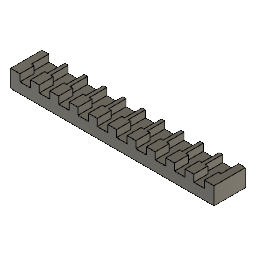
CClampRack3and4in v6 (Autodesk Fusion 360 design; units mm, degrees)
Autodesk Fusion 360 part; units mm, degrees
sketch "Sketch1" plane through (0, 0, 0) normal (0, 0, 1) x (1, 0, 0)
  line L0 (0, 57.15) -> (0, 0)
  line L1 (12.7, 57.15) -> (41.275, 57.15)
  line L2 (41.275, 57.15) -> (41.275, 25.4)
  line L3 (41.275, 25.4) -> (12.7, 25.4)
  line L4 (12.7, 25.4) -> (12.7, 57.15)
  line L5 (26.9875, 25.4) -> (26.9875, 0) construction
  line L6 (17.4625, 25.4) -> (17.4625, 0)
  line L7 (36.5125, 25.4) -> (36.5125, 0)
  line L8 (17.4625, 0) -> (36.5125, 0)
  line L9 (52.3875, 25.4) -> (52.3875, 0)
  line L10 (47.625, 57.15) -> (76.2, 57.15)
  line L11 (61.9125, 25.4) -> (61.9125, 0) construction
  line L12 (47.625, 25.4) -> (47.625, 57.15)
  line L13 (76.2, 25.4) -> (47.625, 25.4)
  line L14 (76.2, 57.15) -> (76.2, 25.4)
  line L15 (71.4375, 25.4) -> (71.4375, 0)
  line L16 (52.3875, 0) -> (71.4375, 0)
  line L17 (87.3125, 25.4) -> (87.3125, 0)
  line L18 (82.55, 57.15) -> (111.125, 57.15)
  line L19 (96.8375, 25.4) -> (96.8375, 0) construction
  line L20 (82.55, 25.4) -> (82.55, 57.15)
  line L21 (111.125, 25.4) -> (82.55, 25.4)
  line L22 (111.125, 57.15) -> (111.125, 25.4)
  line L23 (106.3625, 25.4) -> (106.3625, 0)
  line L24 (87.3125, 0) -> (106.3625, 0)
  line L25 (122.2375, 25.4) -> (122.2375, 0)
  line L26 (117.475, 57.15) -> (146.05, 57.15)
  line L27 (131.7625, 25.4) -> (131.7625, 0) construction
  line L28 (117.475, 25.4) -> (117.475, 57.15)
  line L29 (146.05, 25.4) -> (117.475, 25.4)
  line L30 (146.05, 57.15) -> (146.05, 25.4)
  line L31 (141.2875, 25.4) -> (141.2875, 0)
  line L32 (122.2375, 0) -> (141.2875, 0)
  line L33 (368.3, 57.15) -> (368.3, 0)
  line L34 (368.3, 0) -> (0, 0)
  line L35 (368.3, 57.15) -> (0, 57.15)
  line L36 (176.2125, 25.4) -> (176.2125, 0)
  line L37 (152.4, 57.15) -> (180.975, 57.15)
  line L38 (166.6875, 25.4) -> (166.6875, 0) construction
  line L39 (157.1625, 25.4) -> (157.1625, 0)
  line L40 (180.975, 25.4) -> (152.4, 25.4)
  line L41 (157.1625, 0) -> (176.2125, 0)
  line L42 (180.975, 57.15) -> (180.975, 25.4)
  line L43 (152.4, 25.4) -> (152.4, 57.15)
  line L44 (211.1375, 25.4) -> (211.1375, 0)
  line L45 (187.325, 57.15) -> (215.9, 57.15)
  line L46 (201.6125, 25.4) -> (201.6125, 0) construction
  line L47 (192.0875, 25.4) -> (192.0875, 0)
  line L48 (215.9, 25.4) -> (187.325, 25.4)
  line L49 (192.0875, 0) -> (211.1375, 0)
  line L50 (215.9, 57.15) -> (215.9, 25.4)
  line L51 (187.325, 25.4) -> (187.325, 57.15)
  line L52 (246.0625, 25.4) -> (246.0625, 0)
  line L53 (227.0125, 0) -> (246.0625, 0)
  line L54 (222.25, 57.15) -> (250.825, 57.15)
  line L55 (222.25, 25.4) -> (222.25, 57.15)
  line L56 (227.0125, 25.4) -> (227.0125, 0)
  line L57 (236.5375, 25.4) -> (236.5375, 0) construction
  line L58 (250.825, 25.4) -> (222.25, 25.4)
  line L59 (250.825, 57.15) -> (250.825, 25.4)
  line L60 (280.9875, 25.4) -> (280.9875, 0)
  line L61 (261.9375, 0) -> (280.9875, 0)
  line L62 (257.175, 57.15) -> (285.75, 57.15)
  line L63 (257.175, 25.4) -> (257.175, 57.15)
  line L64 (261.9375, 25.4) -> (261.9375, 0)
  line L65 (271.4625, 25.4) -> (271.4625, 0) construction
  line L66 (285.75, 25.4) -> (257.175, 25.4)
  line L67 (285.75, 57.15) -> (285.75, 25.4)
  line L68 (315.9125, 25.4) -> (315.9125, 0)
  line L69 (296.8625, 0) -> (315.9125, 0)
  line L70 (292.1, 57.15) -> (320.675, 57.15)
  line L71 (292.1, 25.4) -> (292.1, 57.15)
  line L72 (296.8625, 25.4) -> (296.8625, 0)
  line L73 (306.3875, 25.4) -> (306.3875, 0) construction
  line L74 (320.675, 25.4) -> (292.1, 25.4)
  line L75 (320.675, 57.15) -> (320.675, 25.4)
  line L76 (350.8375, 25.4) -> (350.8375, 0)
  line L77 (331.7875, 0) -> (350.8375, 0)
  line L78 (327.025, 57.15) -> (355.6, 57.15)
  line L79 (327.025, 25.4) -> (327.025, 57.15)
  line L80 (331.7875, 25.4) -> (331.7875, 0)
  line L81 (341.3125, 25.4) -> (341.3125, 0) construction
  line L82 (355.6, 25.4) -> (327.025, 25.4)
  line L83 (355.6, 57.15) -> (355.6, 25.4)
  dimension "d2" = 57.15
  dimension "d4" = 28.575
  dimension "d6" = 9.525
  dimension "d7" = 9.525
  dimension "d39" = 31.75
  dimension "d40" = 28.575
  dimension "d41" = 9.525
  dimension "d42" = 9.525
  dimension "d43" = 31.75
  dimension "d44" = 28.575
  dimension "d45" = 9.525
  dimension "d46" = 9.525
  dimension "d47" = 31.75
  dimension "d48" = 28.575
  dimension "d49" = 9.525
  dimension "d50" = 9.525
  dimension "d51" = 31.75
  dimension "d52" = 6.35
  dimension "d53" = 6.35
  dimension "d54" = 6.35
  dimension "d56" = 28.575
  dimension "d57" = 9.525
  dimension "d58" = 9.525
  dimension "d59" = 31.75
  dimension "d60" = 28.575
  dimension "d61" = 9.525
  dimension "d62" = 9.525
  dimension "d63" = 31.75
  dimension "d64" = 6.35
  dimension "d65" = 6.35
  dimension "d77" = 12.7
  dimension "d78" = 28.575
  dimension "d79" = 9.525
  dimension "d80" = 9.525
  dimension "d81" = 31.75
  dimension "d82" = 28.575
  dimension "d83" = 9.525
  dimension "d84" = 9.525
  dimension "d85" = 31.75
  dimension "d86" = 6.35
  dimension "d87" = 6.35
  dimension "d89" = 28.575
  dimension "d90" = 9.525
  dimension "d91" = 9.525
  dimension "d92" = 31.75
  dimension "d93" = 28.575
  dimension "d94" = 9.525
  dimension "d95" = 9.525
  dimension "d96" = 31.75
  dimension "d97" = 12.7
  dimension "d98" = 6.35
  dimension "d99" = 6.35
  measures "d4" distance of L0.end
  measures "d6" distance of L5 L6
  measures "d7" distance of L5 L7
  measures "d41" distance of L9 L11
  measures "d42" distance of L11 L15
  measures "d45" distance of L17 L19
  measures "d46" distance of L19 L23
  measures "d49" distance of L25 L27
  measures "d50" distance of L27 L31
  measures "d52" distance of L2 L12
  measures "d53" distance of L14 L20
  measures "d54" distance of L22 L28
  measures "d57" distance of L38 L39
  measures "d58" distance of L36 L38
  measures "d61" distance of L46 L47
  measures "d62" distance of L44 L46
  measures "d64" distance of L30 L43
  measures "d65" distance of L42 L51
  measures "d77" distance of L0 L4
  measures "d79" distance of L56 L57
  measures "d80" distance of L52 L57
  measures "d83" distance of L64 L65
  measures "d84" distance of L60 L65
  measures "d86" distance of L50 L55
  measures "d87" distance of L59 L63
  measures "d90" distance of L72 L73
  measures "d91" distance of L68 L73
  measures "d94" distance of L80 L81
  measures "d95" distance of L76 L81
  measures "d97" distance of L33 L83
  measures "d98" distance of L67 L71
  measures "d99" distance of L75 L79
extrude "Extrude8" add sketch "Sketch1" against normal blind 31.75
extrude "Extrude9" cut sketch "Sketch1" against normal blind 12.7 contours L1 L2 L3 L4 L35 | L3 L6 L7 L8 L34 | L10 L12 L13 L14 L35 | L9 L13 L15 L16 L34 | L18 L20 L21 L22 L35 | L17 L21 L23 L24 L34 | L26 L28 L29 L30 L35 | L25 L29 L31 L32 L34 | L35 L37 L40 L42 L43 | L34 L36 L39 L40 L41 | L35 L45 L48 L50 L51 | L34 L44 L47 L48 L49 | L35 L54 L55 L58 L59 | L34 L52 L53 L56 L58 | L35 L62 L63 L66 L67 | L34 L60 L61 L64 L66 | L35 L70 L71 L74 L75 | L34 L68 L69 L72 L74 | L35 L78 L79 L82 L83 | L34 L76 L77 L80 L82
